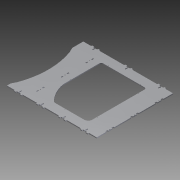
# Autodesk Inventor part: lateral dret
Saved by Autodesk Inventor 2012 SP1 (Build 160190100, 190)
## iProperties
Created: 2014-12-15
Part Number: lateral dret
Material: Default
Document SubType Name: Modeling
Designer: PRINCIPAL
Density: 1 g/cm^3
Author: PRINCIPAL
Autodesk Inventor part; units mm, degrees
ref_plane "YZ Plane" through (0, 0, 0) normal (1, 0, 0) x (0, 1, 0)
ref_plane "XZ Plane" through (0, 0, 0) normal (0, 1, 0) x (-1, 0, 0)
ref_plane "XY Plane" through (0, 0, 0) normal (0, 0, 1) x (1, 0, 0)
sketch "Boceto1" plane through (0, 0, 0) normal (0, 0, 1) x (1, 0, 0)
  line L0 (98.625, 84.15) -> (98.625, 94.05)
  line L1 (98.625, 94.05) -> (103.575, 94.05)
  line L2 (103.575, 94.05) -> (103.575, 84.15)
  line L3 (103.575, 84.15) -> (98.625, 84.15)
  line L4 (98.625, 209.15) -> (98.625, 219.05)
  line L5 (98.625, 219.05) -> (103.575, 219.05)
  line L6 (103.575, 219.05) -> (103.575, 209.15)
  line L7 (103.575, 209.15) -> (98.625, 209.15)
  line L8 (98.625, 334.15) -> (98.625, 344.05)
  line L9 (98.625, 344.05) -> (103.575, 344.05)
  line L10 (103.575, 344.05) -> (103.575, 334.15)
  line L11 (103.575, 334.15) -> (98.625, 334.15)
  line L12 (98.625, 304.15) -> (98.625, 314.05)
  line L13 (98.625, 314.05) -> (103.575, 314.05)
  line L14 (103.575, 314.05) -> (103.575, 304.15)
  line L15 (103.575, 304.15) -> (98.625, 304.15)
  line L16 (98.625, 179.15) -> (98.625, 189.05)
  line L17 (98.625, 189.05) -> (103.575, 189.05)
  line L18 (103.575, 189.05) -> (103.575, 179.15)
  line L19 (103.575, 179.15) -> (98.625, 179.15)
  line L20 (98.625, 54.15) -> (98.625, 64.05)
  line L21 (98.625, 64.05) -> (103.575, 64.05)
  line L22 (103.575, 64.05) -> (103.575, 54.15)
  line L23 (103.575, 54.15) -> (98.625, 54.15)
  arc A0 (453.6069, 72.1) -> (455.6069, 74.1) centre (453.6069, 74.1) ccw
  arc A1 (455.6069, 74.1) -> (453.6069, 76.1) centre (453.6069, 74.1) ccw
  arc A2 (453.6069, 76.1) -> (451.6069, 74.1) centre (453.6069, 74.1) ccw
  arc A3 (451.6069, 74.1) -> (453.6069, 72.1) centre (453.6069, 74.1) ccw
  arc A4 (453.6069, 322.1) -> (455.6069, 324.1) centre (453.6069, 324.1) ccw
  arc A5 (455.6069, 324.1) -> (453.6069, 326.1) centre (453.6069, 324.1) ccw
  arc A6 (453.6069, 326.1) -> (451.6069, 324.1) centre (453.6069, 324.1) ccw
  arc A7 (451.6069, 324.1) -> (453.6069, 322.1) centre (453.6069, 324.1) ccw
  arc A8 (453.6069, 197.1) -> (455.6069, 199.1) centre (453.6069, 199.1) ccw
  arc A9 (455.6069, 199.1) -> (453.6069, 201.1) centre (453.6069, 199.1) ccw
  arc A10 (453.6069, 201.1) -> (451.6069, 199.1) centre (453.6069, 199.1) ccw
  arc A11 (451.6069, 199.1) -> (453.6069, 197.1) centre (453.6069, 199.1) ccw
  arc A12 (101.1, 197.1) -> (103.1, 199.1) centre (101.1, 199.1) ccw
  arc A13 (103.1, 199.1) -> (101.1, 201.1) centre (101.1, 199.1) ccw
  arc A14 (101.1, 201.1) -> (99.1, 199.1) centre (101.1, 199.1) ccw
  arc A15 (99.1, 199.1) -> (101.1, 197.1) centre (101.1, 199.1) ccw
  arc A16 (101.1, 322.1) -> (103.1, 324.1) centre (101.1, 324.1) ccw
  arc A17 (103.1, 324.1) -> (101.1, 326.1) centre (101.1, 324.1) ccw
  arc A18 (101.1, 326.1) -> (99.1, 324.1) centre (101.1, 324.1) ccw
  arc A19 (99.1, 324.1) -> (101.1, 322.1) centre (101.1, 324.1) ccw
  arc A20 (101.1, 72.1) -> (103.1, 74.1) centre (101.1, 74.1) ccw
  arc A21 (103.1, 74.1) -> (101.1, 76.1) centre (101.1, 74.1) ccw
  arc A22 (101.1, 76.1) -> (99.1, 74.1) centre (101.1, 74.1) ccw
  arc A23 (99.1, 74.1) -> (101.1, 72.1) centre (101.1, 74.1) ccw
  line L24 (147.1, 347.0952) -> (357.0956, 347.0952)
  arc A24 (367.0956, 337.0952) -> (357.0956, 347.0952) centre (357.0956, 337.0952) ccw
  line L25 (367.0956, 337.0952) -> (367.0956, 71.1)
  arc A25 (347.0956, 51.1) -> (367.0956, 71.1) centre (347.0956, 71.1) ccw
  line L26 (347.0956, 51.1) -> (200.6723, 51.1)
  arc A26 (186.0973, 57.4043) -> (200.6723, 51.1) centre (200.6723, 71.1) ccw
  arc A27 (137.1, 154.1) -> (186.0973, 57.4043) centre (326.4392, 189.2797) ccw
  line L27 (137.1, 154.1) -> (137.1, 337.0952)
  arc A28 (147.1, 347.0952) -> (137.1, 337.0952) centre (147.1, 337.0952) ccw
  line L28 (172.2133, 393.2) -> (80.2, 393.2)
  line L29 (80.2, 393.2) -> (80.2, 398.2)
  line L30 (80.2, 398.2) -> (69.9334, 398.2)
  line L31 (69.9334, 398.2) -> (69.9334, 393.2)
  line L32 (69.9334, 393.2) -> (62.1933, 393.2)
  line L33 (62.1933, 393.2) -> (62.1933, 387)
  line L34 (62.1933, 387) -> (63.4433, 387)
  line L35 (63.4433, 387) -> (63.4433, 384)
  line L36 (63.4433, 384) -> (62.1933, 384)
  line L37 (62.1933, 384) -> (62.1933, 378.3312)
  line L38 (62.1933, 378.3312) -> (58.1, 378.3312)
  line L39 (58.1, 378.3312) -> (58.1, 384)
  line L40 (58.1, 384) -> (56.85, 384)
  line L41 (56.85, 384) -> (56.85, 387)
  line L42 (56.85, 387) -> (58.1, 387)
  line L43 (58.1, 387) -> (58.1, 393.2)
  line L44 (58.1, 393.2) -> (50.2, 393.2)
  line L45 (50.2, 393.2) -> (50.2, 398.2)
  line L46 (50.2, 398.2) -> (39.9334, 398.2)
  line L47 (39.9334, 398.2) -> (39.9334, 393.2)
  line L48 (39.9334, 393.2) -> (0, 393.2)
  line L49 (0, 393.2) -> (0, 337.9768)
  arc A29 (0, 337.9768) -> (10.9058, 314.7908) centre (173.369, 405.3649) ccw
  arc A30 (10.9058, 45.4092) -> (10.9058, 314.7908) centre (-353.1847, 180.1) ccw
  arc A31 (10.9058, 45.4092) -> (0, 22.2232) centre (133.576, -26.4478) ccw
  line L50 (0, 22.2232) -> (0, 5)
  line L51 (0, 5) -> (40, 5)
  line L52 (40, 5) -> (40, 0)
  line L53 (40, 0) -> (50.2666, 0)
  line L54 (50.2666, 0) -> (50.2666, 5)
  line L55 (50.2666, 5) -> (58.1, 5)
  line L56 (58.1, 5) -> (58.1, 11.2)
  line L57 (58.1, 11.2) -> (56.85, 11.2)
  line L58 (56.85, 11.2) -> (56.85, 14.2)
  line L59 (56.85, 14.2) -> (58.1, 14.2)
  line L60 (58.1, 14.2) -> (58.1, 19.8688)
  line L61 (58.1, 19.8688) -> (62.1933, 19.8688)
  line L62 (62.1933, 19.8688) -> (62.1933, 14.2)
  line L63 (62.1933, 14.2) -> (63.4433, 14.2)
  line L64 (63.4433, 14.2) -> (63.4433, 11.2)
  line L65 (63.4433, 11.2) -> (62.1933, 11.2)
  line L66 (62.1933, 11.2) -> (62.1933, 5)
  line L67 (62.1933, 5) -> (70, 5)
  line L68 (70, 5) -> (70, 0)
  line L69 (70, 0) -> (80.2666, 0)
  line L70 (80.2666, 0) -> (80.2666, 5)
  line L71 (80.2666, 5) -> (152, 5)
  line L72 (152, 5) -> (152, 0)
  line L73 (152, 0) -> (162.2666, 0)
  line L74 (162.2666, 0) -> (162.2666, 5)
  line L75 (162.2666, 5) -> (170.1, 5)
  line L76 (170.1, 5) -> (170.1, 11.2)
  line L77 (170.1, 11.2) -> (168.85, 11.2)
  line L78 (168.85, 11.2) -> (168.85, 14.2)
  line L79 (168.85, 14.2) -> (170.1, 14.2)
  line L80 (170.1, 14.2) -> (170.1, 19.8688)
  line L81 (170.1, 19.8688) -> (174.1933, 19.8688)
  line L82 (174.1933, 19.8688) -> (174.1933, 14.2)
  line L83 (174.1933, 14.2) -> (175.4433, 14.2)
  line L84 (175.4433, 14.2) -> (175.4433, 11.2)
  line L85 (175.4433, 11.2) -> (174.1933, 11.2)
  line L86 (174.1933, 11.2) -> (174.1933, 5)
  line L87 (174.1933, 5) -> (182, 5)
  line L88 (182, 5) -> (182, 0)
  line L89 (182, 0) -> (192.2666, 0)
  line L90 (192.2666, 0) -> (192.2666, 5)
  line L91 (192.2666, 5) -> (264, 5)
  line L92 (264, 5) -> (264, 0)
  line L93 (264, 0) -> (274.2666, 0)
  line L94 (274.2666, 0) -> (274.2666, 5)
  line L95 (274.2666, 5) -> (282.1, 5)
  line L96 (282.1, 5) -> (282.1, 11.2)
  line L97 (282.1, 11.2) -> (280.85, 11.2)
  line L98 (280.85, 11.2) -> (280.85, 14.2)
  line L99 (280.85, 14.2) -> (282.1, 14.2)
  line L100 (282.1, 14.2) -> (282.1, 19.8688)
  line L101 (282.1, 19.8688) -> (286.1933, 19.8688)
  line L102 (286.1933, 19.8688) -> (286.1933, 14.2)
  line L103 (286.1933, 14.2) -> (287.4433, 14.2)
  line L104 (287.4433, 14.2) -> (287.4433, 11.2)
  line L105 (287.4433, 11.2) -> (286.1933, 11.2)
  line L106 (286.1933, 11.2) -> (286.1933, 5)
  line L107 (286.1933, 5) -> (294, 5)
  line L108 (294, 5) -> (294, 0)
  line L109 (294, 0) -> (304.2666, 0)
  line L110 (304.2666, 0) -> (304.2666, 5)
  line L111 (304.2666, 5) -> (376, 5)
  line L112 (376, 5) -> (376, 0)
  line L113 (376, 0) -> (386.2666, 0)
  line L114 (386.2666, 0) -> (386.2666, 5)
  line L115 (386.2666, 5) -> (394.1, 5)
  line L116 (394.1, 5) -> (394.1, 11.2)
  line L117 (394.1, 11.2) -> (392.85, 11.2)
  line L118 (392.85, 11.2) -> (392.85, 14.2)
  line L119 (392.85, 14.2) -> (394.1, 14.2)
  line L120 (394.1, 14.2) -> (394.1, 19.8688)
  line L121 (394.1, 19.8688) -> (398.1933, 19.8688)
  line L122 (398.1933, 19.8688) -> (398.1933, 14.2)
  line L123 (398.1933, 14.2) -> (399.4433, 14.2)
  line L124 (399.4433, 14.2) -> (399.4433, 11.2)
  line L125 (399.4433, 11.2) -> (398.1933, 11.2)
  line L126 (398.1933, 11.2) -> (398.1933, 5)
  line L127 (398.1933, 5) -> (406, 5)
  line L128 (406, 5) -> (406, 0)
  line L129 (406, 0) -> (416.2666, 0)
  line L130 (416.2666, 0) -> (416.2666, 5)
  line L131 (416.2666, 5) -> (456.2, 5)
  line L132 (456.2, 5) -> (456.2, 54.2)
  line L133 (456.2, 54.2) -> (451.2069, 54.2)
  line L134 (451.2069, 54.2) -> (451.2069, 64)
  line L135 (451.2069, 64) -> (456.2, 64)
  line L136 (456.2, 64) -> (456.2, 84.2)
  line L137 (456.2, 84.2) -> (451.2069, 84.2)
  line L138 (451.2069, 84.2) -> (451.2069, 94)
  line L139 (451.2069, 94) -> (456.2069, 94)
  line L140 (456.2069, 94) -> (456.2069, 179.2575)
  line L141 (456.2069, 179.2575) -> (451.2069, 179.2575)
  line L142 (451.2069, 179.2575) -> (451.2069, 189.0575)
  line L143 (451.2069, 189.0575) -> (456.2069, 189.0575)
  line L144 (456.2069, 189.0575) -> (456.2069, 209.2575)
  line L145 (456.2069, 209.2575) -> (451.2069, 209.2575)
  line L146 (451.2069, 209.2575) -> (451.2069, 219.0575)
  line L147 (451.2069, 219.0575) -> (456.2069, 219.0575)
  line L148 (456.2069, 219.0575) -> (456.2069, 304.2)
  line L149 (456.2069, 304.2) -> (451.2069, 304.2)
  line L150 (451.2069, 304.2) -> (451.2069, 314)
  line L151 (451.2069, 314) -> (456.2069, 314)
  line L152 (456.2069, 314) -> (456.2069, 334.2)
  line L153 (456.2069, 334.2) -> (451.2069, 334.2)
  line L154 (451.2069, 334.2) -> (451.2069, 344)
  line L155 (451.2069, 344) -> (456.2, 344)
  line L156 (456.2, 344) -> (456.2, 393.2)
  line L157 (456.2, 393.2) -> (416.2, 393.2)
  line L158 (416.2, 393.2) -> (416.2, 398.2)
  line L159 (416.2, 398.2) -> (405.9334, 398.2)
  line L160 (405.9334, 398.2) -> (405.9334, 393.2)
  line L161 (405.9334, 393.2) -> (398.1933, 393.2)
  line L162 (398.1933, 393.2) -> (398.1933, 387)
  line L163 (398.1933, 387) -> (399.4433, 387)
  line L164 (399.4433, 387) -> (399.4433, 384)
  line L165 (399.4433, 384) -> (398.1933, 384)
  line L166 (398.1933, 384) -> (398.1933, 378.3312)
  line L167 (398.1933, 378.3312) -> (394.1, 378.3312)
  line L168 (394.1, 378.3312) -> (394.1, 384)
  line L169 (394.1, 384) -> (392.85, 384)
  line L170 (392.85, 384) -> (392.85, 387)
  line L171 (392.85, 387) -> (394.1, 387)
  line L172 (394.1, 387) -> (394.1, 393.2)
  line L173 (394.1, 393.2) -> (386.2, 393.2)
  line L174 (386.2, 393.2) -> (386.2, 398.2)
  line L175 (386.2, 398.2) -> (375.9334, 398.2)
  line L176 (375.9334, 398.2) -> (375.9334, 393.2)
  line L177 (375.9334, 393.2) -> (346.9956, 393.2)
  line L178 (346.9956, 393.2) -> (248.2565, 393.2)
  line L179 (248.2565, 393.2) -> (248.2565, 398.2)
  line L180 (248.2565, 398.2) -> (238.0038, 398.2)
  line L181 (238.0038, 398.2) -> (238.0038, 393.2)
  line L182 (238.0038, 393.2) -> (230.1248, 393.2)
  line L183 (230.1248, 393.2) -> (230.1248, 386)
  line L184 (230.1248, 386) -> (231.3718, 386)
  line L185 (231.3718, 386) -> (231.3718, 383)
  line L186 (231.3718, 383) -> (230.1248, 383)
  line L187 (230.1248, 383) -> (230.1248, 377.3312)
  line L188 (230.1248, 377.3312) -> (226.0752, 377.3312)
  line L189 (226.0752, 377.3312) -> (226.0752, 383)
  line L190 (226.0752, 383) -> (224.8282, 383)
  line L191 (224.8282, 383) -> (224.8282, 386)
  line L192 (224.8282, 386) -> (226.0752, 386)
  line L193 (226.0752, 386) -> (226.0752, 393.2)
  line L194 (226.0752, 393.2) -> (218.2197, 393.2)
  line L195 (218.2197, 393.2) -> (218.2197, 398.2)
  line L196 (218.2197, 398.2) -> (207.9729, 398.2)
  line L197 (207.9729, 398.2) -> (207.9729, 393.2)
  line L198 (207.9729, 393.2) -> (172.2133, 393.2)
  point P0 (0, 0)
  constraints: 398 end point, 64 point on circle, 32 centre point
extrude "Extrusión1" add sketch "Boceto1" along normal blind 5
sketch "Boceto2" plane through (0, 0, 5) normal (0, 0, 1) x (1, 0, 0)
  circle A0 centre (370.2069, 304.2) radius 1.25
  circle A1 centre (333.2, 351.2) radius 1.25
  circle A2 centre (171.2, 351.2) radius 1.25
  circle A3 centre (134.2069, 193.2) radius 1.25
  circle A4 centre (251.8392, 49) radius 1.25
  circle A5 centre (370.2069, 96.2) radius 1.25
  line L0 (80.2, 393.2) -> (207.9729, 393.2) projected
  point P0 (0, 0)
  dimension "d8" = 42
  constraints: 6 centre point
  measures "d8" distance from line of point (171.2, 351.2) L0
extrude "Extrusión2" cut sketch "Boceto2" against normal blind 10
